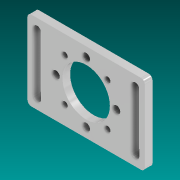
# Autodesk Inventor part: afstandsplaatje
Saved by Autodesk Inventor 2020.2 (Build 242310000, 310)
## iProperties
Created: 2020-05-15
Part Number: afstandsplaatje
Material: Aluminum 6061
Document SubType Name: Modeling
Designer: Svend
Density: 2.7 g/cm^3
Appearance: Aluminum - Polished
Author: Svend
Autodesk Inventor part; units mm, degrees
ref_plane "YZ Plane" through (0, 0, 0) normal (1, 0, 0) x (0, 1, 0)
ref_plane "XZ Plane" through (0, 0, 0) normal (0, 1, 0) x (-1, 0, 0)
ref_plane "XY Plane" through (0, 0, 0) normal (0, 0, 1) x (1, 0, 0)
sketch "Sketch1" plane through (0, 0, 0) normal (0, 0, 1) x (1, 0, 0)
  circle A0 centre (0, 0) radius 21
  circle A1 centre (16, 0) radius 2
  circle A2 centre (0, 16) radius 2
  circle A3 centre (-16, 0) radius 2
  circle A4 centre (0, -16) radius 2
  line L0 (-14.8492, -14.8492) -> (14.8492, 14.8492)
  line L1 (0, -21) -> (0, 21)
  circle A5 centre (11.3137, 11.3137) radius 1.5
  circle A6 centre (-11.3137, 11.3137) radius 1.5
  circle A7 centre (-11.3137, -11.3137) radius 1.5
  circle A8 centre (11.3137, -11.3137) radius 1.5
  circle A9 centre (0, 0) radius 12.6
  line L2 (-21, -21) -> (21, -21)
  line L3 (21, -21) -> (21, 21)
  line L4 (21, 21) -> (-21, 21)
  line L5 (-21, 21) -> (-21, -21)
  line L6 (-21, -21) -> (21, 21) construction
  line L7 (21, -21) -> (-21, 21) construction
  line L8 (-21, 21) -> (-31, 21)
  line L9 (-31, 21) -> (-31, -21)
  line L10 (-31, -21) -> (-21, -21)
  line L11 (-21, -21) -> (-21, 21)
  line L12 (21, 21) -> (31, 21)
  line L13 (31, 21) -> (31, -21)
  line L14 (31, -21) -> (21, -21)
  line L15 (21, -21) -> (21, 21)
  line L16 (-28.1, 17.5) -> (-23.9, 17.5)
  line L17 (-23.9, 17.5) -> (-23.9, -17.5)
  line L18 (-23.9, -17.5) -> (-28.1, -17.5)
  line L19 (-28.1, -17.5) -> (-28.1, 17.5)
  line L20 (-28.1, 17.5) -> (-23.9, -17.5) construction
  line L21 (-23.9, 17.5) -> (-28.1, -17.5) construction
  line L22 (23.9, 17.5) -> (28.1, 17.5)
  line L23 (28.1, 17.5) -> (28.1, -17.5)
  line L24 (28.1, -17.5) -> (23.9, -17.5)
  line L25 (23.9, -17.5) -> (23.9, 17.5)
  line L26 (23.9, 17.5) -> (28.1, -17.5) construction
  line L27 (28.1, 17.5) -> (23.9, -17.5) construction
  point P0 (-18.984, 8.9782)
  point P1 (-18.984, -8.9782)
  point P2 (-26, 0)
  point P3 (26, 0)
  point P4 (-26, 0)
  point P5 (26, 0)
  point P6 (26, 0)
  point P7 (26, 21)
  point P8 (-26, 0)
  point P9 (-26, 21)
  dimension "d0" = 42
  dimension "d1" = 4
  dimension "d5" = 16
  dimension "d8" = 360
  dimension "d10" = 45
  dimension "d11" = 3
  dimension "d12" = 16
  dimension "d15" = 360
  dimension "d19" = 25.2
  dimension "d30" = 10
  dimension "d31" = 4.2
  dimension "d32" = 35
  dimension "d33" = 4.2
  constraints: 56 end point, 18 midpoint, 10 centre point, 10 parallel, 6 point on circle, 5 horizontal, 5 perpendicular, 3 collinear, 3 horizontal alignment, 2 coincident, 2 point on line, 2 tangent, 2 vertical alignment, 1 vertical, 18 other
  measures "d0" diameter of A0
  measures "d1" diameter of A1
  measures "d5" distance of point (0, 0) A1.centre
  measures "d10" angle of L1 L0
  measures "d11" diameter of A5
  measures "d12" distance of point (0, 0) A5.centre
  measures "d19" diameter of A9
  measures "d30" distance of L10.end L9.end
  measures "d31" distance of L17.end L18.end
  measures "d32" distance of L16.end L17.end
  measures "d33" distance of L23.end L24.end
extrude "Extrusion1" add sketch "Sketch1" along normal blind 4 contours A0 L1 A4 A9 L0 A5 | L3 L2 A0 | L3 L12 L13 L14 | A0 L4 L3 | L0 A5 A9 L1 A2 A0 | L2 L5 A0 | A0 L0 A7 A9 L1 A4 | L1 A2 A9 L0 A7 A0 | A0 L5 L4 | L10 L9 L8 L5
fillet "Fillet1" radius 2 4 edges at (-31, 21, 2) (-31, -21, 2) (31, -21, 2) (31, 21, 2)
fillet "Fillet2" radius 2.1 8 edges at (28.1, -17.5, 2) (23.9, -17.5, 2) (23.9, 17.5, 2) (28.1, 17.5, 2) (-28.1, 17.5, 2) (-23.9, 17.5, 2) (-23.9, -17.5, 2) (-28.1, -17.5, 2)
body "Solid1"
